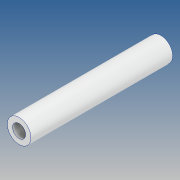
# Autodesk Inventor part: 104.005.01_Distanzbuchse
Saved by Autodesk Inventor 2021 (Build 250183000, 183)
## iProperties
Created: 2021-12-03
Part Number: 104.005.01_Distanzbuchse
Material: Aluminium 6061
Document SubType Name: Modeling
Designer: Oliver Ungerer
Density: 2.7 g/cm^3
Appearance: Aluminium - flach
Mass: 8.87461 g
Surface Area: 30.3124 cm^2
Volume: 3.28689 cm^3
Author: Oliver Ungerer
Title: Distanzbuchse
Autodesk Inventor part; units mm, degrees
ref_plane "YZ Plane" through (0, 0, 0) normal (1, 0, 0) x (0, 1, 0)
ref_plane "XZ Plane" through (0, 0, 0) normal (0, 1, 0) x (-1, 0, 0)
ref_plane "XY Plane" through (0, 0, 0) normal (0, 0, 1) x (1, 0, 0)
sketch "Skizze1" plane through (0, 0, 0) normal (0, 0, 1) x (1, 0, 0)
  circle A0 centre (0, 0) radius 2.75
  circle A1 centre (0, 0) radius 5
  dimension "d0" = 5.5
  dimension "d1" = 10
  constraints: 2 centre point, 2 coincident
  measures "d0" diameter of A0
  measures "d1" diameter of A1
extrude "Extrusion1" add sketch "Skizze1" along normal blind 60
